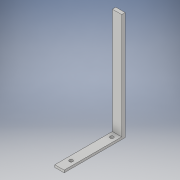
# Autodesk Inventor part: soporte3pantalla
Saved by Autodesk Inventor 2019 (Build 230136000, 136)
## iProperties
Created: 2019-03-07
Part Number: soporte3pantalla
Material: Genérico
Document SubType Name: Modeling
Designer: flakt
Density: 1 g/cm^3
Appearance: Valor por defecto
Author: flakt
Autodesk Inventor part; units mm, degrees
ref_plane "YZ Plane" through (0, 0, 0) normal (1, 0, 0) x (0, 1, 0)
ref_plane "XZ Plane" through (0, 0, 0) normal (0, 1, 0) x (-1, 0, 0)
ref_plane "XY Plane" through (0, 0, 0) normal (0, 0, 1) x (1, 0, 0)
sketch "Boceto1" plane through (0, 0, 0) normal (0, 1, 0) x (-1, 0, 0)
  line L0 (112.646, 23.1115) -> (33.646, 23.1115)
  circle A0 centre (89.8586, 65.5785) radius 1.5
  circle A1 centre (89.8586, 65.5785) radius 1.5
  circle A2 centre (103.0678, 65.5785) radius 1.5
  line L1 (103.0678, 65.5785) -> (103.0678, 30.5785)
  circle A3 centre (103.0678, 30.5785) radius 1.5
  line L2 (103.0678, 30.5785) -> (99.0678, 30.5785)
  line L3 (99.0678, 30.5785) -> (99.0678, 25.5785)
  line L4 (99.0678, 25.5785) -> (107.0678, 25.5785)
  line L5 (107.0678, 25.5785) -> (107.0678, 75.5785)
  line L6 (107.0678, 75.5785) -> (99.0678, 75.5785)
  line L7 (99.0678, 75.5785) -> (99.0678, 25.5785)
  point P0 (0, 0)
  dimension "d0" = 35
  dimension "d1" = 3
  dimension "d2" = 4
  dimension "d3" = 5
  dimension "d4" = 8
  dimension "d5" = 50
  constraints: 16 end point, 4 centre point, 2 coincident, 2 horizontal, 2 parallel, 2 vertical, 1 concentric, 1 perpendicular
  measures "d0" distance of L1.start L1.end
  measures "d1" diameter of A3
  measures "d2" distance of L2.start L2.end
  measures "d3" distance of L2.end L3.end
  measures "d4" distance of L6.end L5.end
  measures "d5" distance of L5.end L4.end
extrude "Extrusión1" add sketch "Boceto1" along normal blind 2 contours L7 L6 L5 L4 L3
thicken "Engrosado1" operation add thickness 2.467 both sides no extend neighbours yes toward (0, 0, -1) faces at (-101.7345, 0.6667, 25.5785)
sketch "Boceto2" plane through (0, 2, 0) normal (0, 1, 0) x (1, 0, 0)
  line L0 (-99.0678, -23.1115) -> (-107.0678, -23.1115) projected
  line L1 (-99.0678, -75.5785) -> (-99.0678, -23.1115) projected
  line L2 (-107.0678, -23.1115) -> (-99.0678, -23.1115)
  line L3 (-99.0678, -23.1115) -> (-99.0678, -26.1115)
  line L4 (-99.0678, -26.1115) -> (-107.0678, -26.1115)
  line L5 (-107.0678, -26.1115) -> (-107.0678, -23.1115)
  point P0 (0, 0)
  dimension "d10" = 3
  constraints: 8 end point, 2 parallel, 1 horizontal, 1 perpendicular, 1 point on line
  measures "d10" distance of L2.end L3.end
extrude "Extrusión2" add sketch "Boceto2" along normal blind 91
